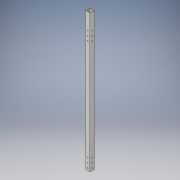
# Autodesk Inventor part: 30in 1x1 Beam
Saved by Autodesk Inventor 2018 (Build 220112000, 112)
## iProperties
Created: 2019-01-16
Part Number: 30in 1x1 Beam
Material: Generic
Document SubType Name: Modeling
Designer: Gabriel
Density: 1 g/cm^3
Appearance: Default
Author: Gabriel
Autodesk Inventor part; units mm, degrees
ref_plane "YZ Plane" through (0, 0, 0) normal (1, 0, 0) x (0, 1, 0)
ref_plane "XZ Plane" through (0, 0, 0) normal (0, 1, 0) x (-1, 0, 0)
ref_plane "XY Plane" through (0, 0, 0) normal (0, 0, 1) x (1, 0, 0)
sketch "Sketch1" plane through (0, 0, 0) normal (0, 1, 0) x (-1, 0, 0)
  line L0 (2.2807, -2.5252) -> (-23.1193, -2.5252)
  line L1 (-23.1193, -2.5252) -> (-23.1193, 22.8748)
  line L2 (-23.1193, 22.8748) -> (2.2807, 22.8748)
  line L3 (2.2807, 22.8748) -> (2.2807, -2.5252)
  line L4 (-19.9443, 0.6498) -> (-0.8943, 0.6498)
  line L5 (-0.8943, 0.6498) -> (-0.8943, 19.6998)
  line L6 (-0.8943, 19.6998) -> (-19.9443, 19.6998)
  line L7 (-19.9443, 19.6998) -> (-19.9443, 0.6498)
  point P0 (0, 0)
  dimension "d0" = 25.4
  dimension "d1" = 25.4
  dimension "d2" = 3.175
  constraints: 16 end point, 4 parallel, 2 perpendicular, 1 horizontal, 3 other
  measures "d0" distance of L1.end L2.end
  measures "d1" distance of L0.end L1.end
  measures "d2" distance between parallel lines of L0 L4
extrude "Extrusion1" add sketch "Sketch1" along normal blind 762
sketch "Sketch2" plane through (-2.2807, 0, -2.5252) normal (-1, 0, 0) x (0, 0, 1)
  line L0 (25.4, 762) -> (0, 762) projected
  line L1 (22.225, 0) -> (3.175, 0) projected
  circle A0 centre (12.7, 12.7) radius 2.5797
  line L2 (12.7, 12.7) -> (12.7, 38.1) construction
  line L3 (12.7, 38.1) -> (12.7, 63.5) construction
  circle A1 centre (12.7, 63.5) radius 2.5797
  circle A2 centre (12.7, 38.1) radius 2.5797
  line L4 (12.7, 12.7) -> (12.7, 0) construction
  line L5 (12.7, 762) -> (12.7, 635) construction
  circle A3 centre (12.7, 673.1) radius 2.5797
  line L6 (12.7, 673.1) -> (12.7, 647.7) construction
  line L7 (12.7, 647.7) -> (12.7, 622.3) construction
  circle A4 centre (12.7, 647.7) radius 2.5797
  circle A5 centre (12.7, 622.3) radius 2.5797
  point P0 (2.5252, 0)
  dimension "d8" = 5.1594
  dimension "d9" = 25.4
  dimension "d10" = 25.4
  dimension "d11" = 5.1594
  dimension "d12" = 5.1594
  dimension "d33" = 5.1594
  dimension "d34" = 25.4
  dimension "d35" = 25.4
  dimension "d36" = 5.1594
  dimension "d37" = 5.1594
  constraints: 12 end point, 6 centre point, 4 coincident, 3 vertical, 2 midpoint, 2 point on line
  measures "d8" diameter of A0
  measures "d9" distance of L2.start L2.end
  measures "d10" distance of L2.end L3.end
  measures "d11" diameter of A1
  measures "d12" diameter of A2
  measures "d33" diameter of A3
  measures "d34" distance of L6.start L6.end
  measures "d35" distance of L6.end L7.end
  measures "d36" diameter of A4
  measures "d37" diameter of A5
extrude "Extrusion2" cut sketch "Sketch2" against normal blind 762
sketch "Sketch3" plane through (-2.2807, 0, 22.8748) normal (0, 0, 1) x (1, 0, 0)
  line L0 (22.225, 0) -> (3.175, 0) construction
  line L1 (12.7, 0) -> (12.7, 12.7) construction
  line L2 (12.7, 12.7) -> (12.7, 38.1) construction
  line L3 (12.7, 38.1) -> (12.7, 63.5) construction
  circle A0 centre (12.7, 63.5) radius 2.5797
  circle A1 centre (12.7, 38.1) radius 2.5797
  circle A2 centre (12.7, 12.7) radius 2.5797
  line L4 (12.7, 685.8) -> (12.7, 673.1) construction
  circle A3 centre (12.7, 673.1) radius 2.5797
  line L5 (12.7, 673.1) -> (12.7, 647.7) construction
  line L6 (12.7, 647.7) -> (12.7, 622.3) construction
  circle A4 centre (12.7, 647.7) radius 2.5797
  circle A5 centre (12.7, 622.3) radius 2.5797
  point P0 (2.2807, 0)
  dimension "d19" = 12.7
  dimension "d20" = 25.4
  dimension "d21" = 25.4
  dimension "d22" = 5.1594
  dimension "d23" = 5.1594
  dimension "d24" = 5.1594
  dimension "d38" = 12.7
  dimension "d39" = 5.1594
  dimension "d40" = 25.4
  dimension "d41" = 25.4
  dimension "d42" = 5.1594
  dimension "d43" = 5.1594
  constraints: 12 end point, 6 centre point, 6 coincident, 3 point on line, 2 vertical, 1 midpoint
  measures "d19" distance of L1.start L1.end
  measures "d20" distance of L1.end L2.end
  measures "d21" distance of L2.end L3.end
  measures "d22" diameter of A0
  measures "d23" diameter of A1
  measures "d24" diameter of A2
  measures "d38" distance of L4.start L4.end
  measures "d39" diameter of A3
  measures "d40" distance of L5.start L5.end
  measures "d41" distance of L5.end L6.end
  measures "d42" diameter of A4
  measures "d43" diameter of A5
extrude "Extrusion3" cut sketch "Sketch3" against normal blind 762
body "Solid1"
